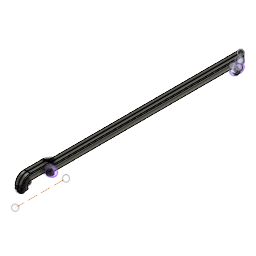
pret_1 (Autodesk Fusion 360 design; units mm, degrees)
part number: 2026-01-04-18-27-24-401
Autodesk Fusion 360 part; units mm, degrees
note: some values were not read from the file. Set by a fixed rule: which sketch regions a step uses.
sketch "Szkic1" plane through (0, 0, 0) normal (1, 0, 0) x (0, 1, 0)
  line L0 (-2.5, 0.8) -> (-2.5, 3)
  line L1 (4.5, 10) -> (19.5, 10)
  line L2 (17.4289, 5) -> (4.5, 5)
  line L3 (2.5, 3) -> (2.5, 0.8)
  line L4 (1.7, 0) -> (-1.7, 0)
  arc A0 (-2.5, 0.8) -> (-1.7, 0) centre (-1.7, 0.8) ccw
  arc A1 (1.7, 0) -> (2.5, 0.8) centre (1.7, 0.8) ccw
  arc A2 (4.5, 10) -> (-2.5, 3) centre (4.5, 3) ccw
  arc A3 (4.5, 5) -> (2.5, 3) centre (4.5, 3) ccw
  line L5 (17.7825, 4.8536) -> (20.3431, 2.2929)
  line L6 (22.4142, 7.2929) -> (19.8536, 9.8536)
  line L7 (172.2071, 7) -> (23.1213, 7)
  line L8 (21.0503, 2) -> (166.2071, 2)
  line L9 (172.7071, 2.5) -> (172.7071, 6.5)
  arc A4 (19.8536, 9.8536) -> (19.5, 10) centre (19.5, 9.5) ccw
  arc A5 (17.7825, 4.8536) -> (17.4289, 5) centre (17.4289, 4.5) ccw
  arc A6 (22.4142, 7.2929) -> (23.1213, 7) centre (23.1213, 8) ccw
  arc A7 (172.7071, 6.5) -> (172.2071, 7) centre (172.2071, 6.5) ccw
  arc A8 (172.2071, 2) -> (172.7071, 2.5) centre (172.2071, 2.5) ccw
  arc A9 (20.3431, 2.2929) -> (21.0503, 2) centre (21.0503, 3) ccw
  line L10 (166.7071, 1.5) -> (166.7071, -2.2)
  line L11 (167.5071, -3) -> (170.9071, -3)
  line L12 (171.7071, -2.2) -> (171.7071, 1.5)
  arc A10 (172.2071, 2) -> (171.7071, 1.5) centre (172.2071, 1.5) ccw
  arc A11 (166.7071, 1.5) -> (166.2071, 2) centre (166.2071, 1.5) ccw
  arc A12 (166.7071, -2.2) -> (167.5071, -3) centre (167.5071, -2.2) ccw
  arc A13 (170.9071, -3) -> (171.7071, -2.2) centre (170.9071, -2.2) ccw
  line L13 (-5, -10) -> (35, -10) construction
  point P0 (172.7071, 7)
  dimension "d9" = 0.8
  dimension "d10" = 0.8
  dimension "d14" = 5
  dimension "d16" = 135
  dimension "d17" = 5
  dimension "d21" = 0.5
  dimension "d24" = 0.5
  dimension "d25" = 0.5
  dimension "d28" = 15
  dimension "d37" = 1
  dimension "d39" = 1
  dimension "d71" = 0.5
  dimension "d73" = 5
  dimension "d75" = 0.5
  dimension "d79" = 0.8
  dimension "d80" = 0.8
  dimension "d84" = 5
  dimension "d86" = 2
  dimension "d87" = 10
  dimension "d88" = 2
  dimension "d89" = 5
  dimension "d91" = 1
  dimension "d101" = 171.7071
  constraint vertical L0
  constraint perpendicular L0 L1
  constraint perpendicular L1 L3
  constraint perpendicular L0 L4
  constraint tangent L0 A0
  constraint tangent L4 A0
  constraint tangent L4 A1
  constraint tangent L3 A1
  constraint tangent L1 A2
  constraint tangent L0 A2
  constraint tangent L3 A3
  constraint tangent L2 A3
  constraint concentric A2 A3
  constraint perpendicular L7 L9
  constraint tangent L1 A4
  constraint tangent L6 A4
  constraint tangent L2 A5
  constraint tangent L5 A5
  constraint equal A4 A5
  constraint tangent L6 A6
  constraint tangent L7 A6
  constraint coincident P0 L7
  constraint coincident P0 L9
  constraint tangent L7 A7
  constraint tangent L9 A7
  constraint tangent L8 A8
  constraint tangent L9 A8
  constraint parallel L2 L8
  constraint horizontal L7
  constraint tangent L8 A9
  constraint tangent L5 A9
  constraint midpoint L4 origin
  constraint vertical L10
  constraint horizontal L11
  constraint vertical L12
  constraint tangent A8 A10
  constraint tangent L12 A10
  constraint tangent L8 A11
  constraint tangent L10 A11
  constraint tangent L10 A12
  constraint tangent L11 A12
  constraint tangent L11 A13
  constraint tangent L12 A13
  constraint horizontal L13
  measures "d9" radius of A0
  measures "d10" radius of A1
  measures "d14" distance of L5 L6
  measures "d16" angle of L6 L7
  measures "d17" distance of L7 L8
  measures "d21" radius of A4
  measures "d24" radius of A7
  measures "d25" radius of A8
  measures "d28" distance of L1.start L1.end
  measures "d37" radius of A9
  measures "d39" radius of A6
  measures "d71" radius of A10
  measures "d73" distance of L8 L11
  measures "d75" radius of A11
  measures "d79" radius of A12
  measures "d80" radius of A13
  measures "d84" distance of A2 A3
  measures "d86" radius of A3
  measures "d87" distance of L1 L4
  measures "d88" distance of L4 L8
  measures "d89" distance of L10 L12
  measures "d91" distance of L9 L12
  measures "d101" distance of origin L12
extrude "Wyciągnięcie proste1" add sketch "Szkic1" along normal mid plane 6
sketch "Szkic2" plane through (0, 0, 0) normal (1, 0, 0) x (0, 1, 0)
  line L0 (0, -2.8) -> (0, 0.6)
  arc A0 (0, -2.8) -> (0, 0.6) centre (0, -1.1) ccw
  dimension "d30" = 3.4
  dimension "d41" = 1.1
  constraint vertical L0
  constraint midpoint A0.centre L0
  constraint coincident origin L0
  measures "d30" diameter of A0
  measures "d41" distance of origin A0.centre
fillet "Zaokrąglenie1" radius 0.5 20 edges at (3, 2.5, 1.9) (3, 3.0858, 4.4142) (3, 10.9645, 5) (3, 17.6203, 4.9619) (3, 19.0628, 3.5732) (3, 20.6676, 2.0761) (3, 93.6287, 2) (3, 172.5607, 2.1464) (3, 172.7071, 4.5) (3, 172.5607, 6.8536) (3, 97.6642, 7) (3, 22.7386, 7.0761) (3, 21.1339, 8.5732) (3, 19.6913, 9.9619) (3, 12, 10) (3, -0.4497, 7.9497) (3, -2.5, 1.9) (3, -2.2657, 0.2343) (3, 0, 0) (3, 2.2657, 0.2343)
fillet "Zaokrąglenie2" radius 0.5 20 edges at (-3, -2.5, 1.9) (-3, -0.4497, 7.9497) (-3, 12, 10) (-3, 19.6913, 9.9619) (-3, 21.1339, 8.5732) (-3, 22.7386, 7.0761) (-3, 97.6642, 7) (-3, 172.5607, 6.8536) (-3, 172.7071, 4.5) (-3, 172.5607, 2.1464) (-3, 93.6287, 2) (-3, 20.6676, 2.0761) (-3, 19.0628, 3.5732) (-3, 17.6203, 4.9619) (-3, 10.9645, 5) (-3, 3.0858, 4.4142) (-3, 2.5, 1.9) (-3, 2.2657, 0.2343) (-3, 0, 0) (-3, -2.2657, 0.2343)
revolve "Obrót1" add sketch "Szkic2" angle 360 about axis through (0, 0, 1.75) along (0, 0, 1)
sketch "Szkic3" plane through (0, 0, 0) normal (1, 0, 0) x (0, 1, 0)
  arc A0 (24.6651, -0.75) -> (22.5, 3) centre (22.5, 0.5) ccw
  line L0 (22.5, -0.75) -> (22.5, 3)
  line L1 (24.6651, -0.75) -> (22.5, -0.75)
  line L2 (22.5, 3) -> (22.5, 0.5) construction
  dimension "d33" = 5
  dimension "d43" = 1.25
  dimension "d44" = 22.5
  dimension "d92" = 0.5
  constraint horizontal L1
  constraint coincident A0.centre L2.end
  constraint vertical L2
  constraint vertical L0
  measures "d33" diameter of A0
  measures "d43" distance of A0.centre L1
  measures "d44" horizontal distance of origin A0.centre
  measures "d92" vertical distance of origin A0.centre
revolve "Obrót2" cut sketch "Szkic3" angle 360 about axis through (0, 22.5, -0.75) along (0, 0, 1)
revolve "Obrót3" add sketch "Szkic3" angle 360 about axis through (0, 22.5, 3) along (0, 0, -1)
sketch "Szkic4" plane through (3, 0, 0) normal (1, 0, 0) x (0, 1, 0)
  line L0 (22.25, -0.75) -> (22.75, -0.75)
  line L1 (22.75, -0.75) -> (22.75, 0.5)
  line L2 (22.75, 0.5) -> (22.25, 0.5)
  line L3 (22.25, 0.5) -> (22.25, -0.75)
  line L4 (2, 0.8) -> (2, 3)
  arc A0 (4.5, 5.5) -> (2, 3) centre (4.5, 3) ccw
  line L5 (4.5, 5.5) -> (17.4289, 5.5)
  arc A1 (18.136, 5.2071) -> (17.4289, 5.5) centre (17.4289, 4.5) ccw
  line L6 (18.136, 5.2071) -> (20.6967, 2.6464)
  arc A2 (20.6967, 2.6464) -> (21.0503, 2.5) centre (21.0503, 3) ccw
  line L7 (21.0503, 2.5) -> (166.2071, 2.5)
  line L8 (172.2071, 2.5) -> (172.2071, 6.5)
  line L9 (172.2071, 6.5) -> (23.1213, 6.5)
  arc A3 (22.0607, 6.9393) -> (23.1213, 6.5) centre (23.1213, 8) ccw
  line L10 (22.0607, 6.9393) -> (19.5, 9.5)
  line L11 (19.5, 9.5) -> (4.5, 9.5)
  arc A4 (4.5, 9.5) -> (-2, 3) centre (4.5, 3) ccw
  line L12 (-2, 3) -> (-2, 0.8)
  arc A5 (-2, 0.8) -> (-1.7, 0.5) centre (-1.7, 0.8) ccw
  line L13 (-1.7, 0.5) -> (1.7, 0.5)
  arc A6 (1.7, 0.5) -> (2, 0.8) centre (1.7, 0.8) ccw
  line L14 (171.2071, -2.2) -> (171.2071, 1.5)
  arc A7 (172.2071, 2.5) -> (171.2071, 1.5) centre (172.2071, 1.5) ccw
  arc A8 (167.2071, 1.5) -> (166.2071, 2.5) centre (166.2071, 1.5) ccw
  line L15 (167.2071, 1.5) -> (167.2071, -2.2)
  arc A9 (167.2071, -2.2) -> (167.5071, -2.5) centre (167.5071, -2.2) ccw
  line L16 (167.5071, -2.5) -> (170.9071, -2.5)
  arc A10 (170.9071, -2.5) -> (171.2071, -2.2) centre (170.9071, -2.2) ccw
  point P0 (22.5, -0.75)
  dimension "d47" = 0.5
  dimension "d48" = 1.25
  dimension "d49" = 22.75
  constraint horizontal L0
  constraint vertical L1
  constraint horizontal L2
  constraint vertical L3
  constraint coincident L0 P0
  measures "d47" distance of L0.start L0.end
  measures "d48" distance of L0.end L1.end
  measures "d49" horizontal distance of origin L0.end
extrude "Wyciągnięcie proste2" cut sketch "Szkic4" along normal mid plane 20 contours L0 L1 L2 L3
pattern_circular "Szyk kołowy1" count 4 over 360 about axis through (0, 22.5, 3) along (0, 0, -1) of "Wyciągnięcie proste2"
fillet "Zaokrąglenie4" radius 0.25 2 edges at (0, 24.5, 2) (0, 20.5895, 2.1125)
sketch "Szkic6" plane through (0, 0, 0) normal (1, 0, 0) x (0, 1, 0)
  line L0 (169.2071, -2.4) -> (169.2071, -5.8)
  arc A0 (169.2071, -5.8) -> (169.2071, -2.4) centre (169.2071, -4.1) ccw
  line L1 (167.5071, -3) -> (170.9071, -3)
  line L2 (171.7071, -2.2) -> (171.7071, 1.5)
  dimension "d67" = 3.4
  dimension "d96" = 1.1
  dimension "d104" = 2.5
  constraint vertical L0
  constraint coincident A0.centre L0
  measures "d67" diameter of A0
  measures "d96" distance of A0.centre L1
  measures "d104" distance of L0 L2
revolve "Obrót4" add sketch "Szkic6" angle 360 about axis through (0, 169.2071, -2.4) along (0, 0, -1)
fillet "Zaokrąglenie6" radius 0.5 1 edges at (-0.4687, 170.4155, -3)
fillet "Zaokrąglenie7" radius 0.5 1 edges at (-0.4687, 1.2084, 0)
sketch "Szkic7" plane through (0, 0, 0) normal (1, 0, 0) x (0, 1, 0)
  arc A0 (24.6651, -0.75) -> (22.5, 3) centre (22.5, 0.5) ccw
  line L0 (22.5, 2.25) -> (22.5, -1.25)
  arc A1 (22.5, -1.25) -> (22.5, 2.25) centre (22.5, 0.5) ccw
  dimension "d102" = 3.5
  constraint concentric A0 A1
  constraint vertical L0
  constraint coincident A0.centre L0
  measures "d102" diameter of A1
revolve "Obrót5" cut sketch "Szkic7" angle 360 about axis through (0, 22.5, 2.25) along (0, 0, -1)
